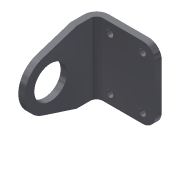
# Autodesk Inventor part: cyl mount
Saved by Autodesk Inventor 2022 Beta2 (Build 260130000, 130) ContinuousBuild 0
## iProperties
Shininess: 60.0
Length Units: 11272
Angle Units: 11279
Time Units: 11290
Mass Units: 11286
Length Display Precision: 3
Angle Display Precision: 2
Created: 2001-07-19
Part Number: cyl mount
Document SubType Name: Sheet Metal
Designer: smithga
Density: 1 g/cm^3
Sheet Metal Rule: Default
Material: Generic
Appearance: Metal-Steel(Polish)
Density: 0.0
Volumn: 0.0
Area: 0.0
PropertySet Name: Model Information
Control State: 0
Master: False
Checked Out: False
Author: smithga
Autodesk Inventor part; units mm, degrees
ref_plane "YZ Plane" through (0, 0, 0) normal (1, 0, 0) x (0, 1, 0)
ref_plane "XZ Plane" through (0, 0, 0) normal (0, 1, 0) x (-1, 0, 0)
ref_plane "XY Plane" through (0, 0, 0) normal (0, 0, 1) x (1, 0, 0)
sketch "Sketch1" plane through (0, 0, 0) normal (0, 0, 1) x (1, 0, 0)
  line L0 (-63.5, 22.225) -> (-31.75, 22.225)
  line L1 (-31.75, 22.225) -> (-31.75, -12.7)
  line L2 (-31.75, -12.7) -> (-63.5, -12.7)
  line L3 (-63.5, -12.7) -> (-63.5, 22.225)
extrude "Plate1" add sketch "Sketch1" along normal blind 3.048
sketch "Sketch2" plane through (-63.5, 22.225, 3.048) normal (0, 0, 1) x (1, 0, 0)
  circle A0 centre (9.525, -4.7821) radius 1.651 projected
  circle A1 centre (25.4, -4.7821) radius 1.651 projected
  circle A2 centre (9.525, -30.1821) radius 1.651 projected
  circle A3 centre (25.4, -30.1821) radius 1.651 projected
extrude "Cut1" cut sketch "Sketch2" against normal through all
sketch "Sketch3" plane through (-63.5, 22.225, 0) normal (1, 0, 0) x (0, -1, 0)
  line L0 (0, 0) -> (34.925, 0)
  line L1 (34.925, 0) -> (34.925, -38.1)
  line L2 (34.925, -38.1) -> (0, -38.1)
  line L3 (0, -38.1) -> (0, 0)
  constraints: 4 end point, 4 other
sheet face with bend "Flange1" sketch "Sketch3" thickness 3.048 toward (1, 0, 0) bend radius 3.048 relief straight relief width 3.048 relief depth 1.524
bend "Bend1"
sketch "Sketch4" plane through (-63.5, -12.7, 38.1) normal (-1, 0, 0) x (0, 0, 1)
  line L0 (-32.004, 0) -> (0, 0) projected
  line L1 (0, 0) -> (0, 34.925) projected
  line L2 (0, 34.925) -> (-32.004, 34.925) projected
  line L3 (0, 17.4625) -> (-12.7, 17.4625) construction
  line L4 (-12.7, 17.4625) -> (-12.7, 34.925) construction
  arc A0 (-8.787, 5.3803) -> (-8.787, 29.5447) centre (-12.7, 17.4625) ccw
  line L5 (-25.4, 34.925) -> (-8.787, 29.5447)
  line L6 (-25.4, 0) -> (-8.787, 5.3803)
  circle A1 centre (-12.7, 17.4625) radius 7.9375
  constraints: 8 end point, 3 point on circle, 3 point on line, 2 centre point, 2 coincident, 2 tangent, 1 midpoint, 1 parallel, 1 perpendicular
extrude "Cut2" cut sketch "Sketch4" against normal through all
fillet "Corner Round1" radius 6.35 2 edges at (-31.75, 22.225, 1.524) (-31.75, -12.7, 1.524)
equation "\"d1\" = Thickness"
equation "\"d7\" = Thickness"
equation "\"d13\" = Thickness"
equation "\"d6\" = BendRadius"
equation "\"MinimumRemnant\" = 2 * Thickness"
equation "\"BendReliefWidth\" = Thickness"
equation "\"d3\" = BendRadius"
equation "\"d10\" = BendReliefWidth"
equation "\"d11\" = BendReliefDepth"
equation "\"d12\" = MinimumRemnant"
equation "\"BendRadius\" = Thickness"
equation "\"BendReliefDepth\" = 0.5 * Thickness"
equation "\"CornerReliefSize\" = 4 * Thickness"
equation "\"TransitionRadius\" = BendRadius"
equation "\"d0\" = BendRadius"
equation "\"JacobiRadiusSize\" = Thickness"
equation "\"GapSize\" = Thickness"
equation "\"Thickness\" = 3.048"
body "Solid1"
